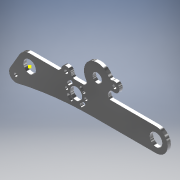
# Autodesk Inventor part: Intake Arm
Saved by Autodesk Inventor 2019.4 (Build 234330000, 330)
## iProperties
Created: 2020-01-28
Part Number: Intake Arm
Material: Aluminum 6061
Document SubType Name: Modeling
Designer: admin
Density: 2.7 g/cm^3
Appearance: Aluminum - Flat
Mass: 119.652 g
Surface Area: 228.427 cm^2
Volume: 44.3155 cm^3
Author: admin
Autodesk Inventor part; units mm, degrees
ref_plane "YZ Plane" through (0, 0, 0) normal (1, 0, 0) x (0, 1, 0)
ref_plane "XZ Plane" through (0, 0, 0) normal (0, 1, 0) x (-1, 0, 0)
ref_plane "XY Plane" through (0, 0, 0) normal (0, 0, 1) x (1, 0, 0)
sketch "Sketch1" plane through (0, 0, 0) normal (0, 0, 1) x (1, 0, 0)
  circle A0 centre (0, 0) radius 9.5
  arc A1 (0, -17.5) -> (0, 17.5) centre (0, 0) ccw construction
  circle A2 centre (190, 0) radius 9.5
  circle A3 centre (-175.4753, -121.2237) radius 88.9 construction
  circle A4 centre (190, 0) radius 41.275 construction
  circle A5 centre (190, 0) radius 28.5 construction
  line L0 (-263.1536, 888.7662) -> (-263.1536, -773.9924) construction
  line L1 (0, 0) -> (190, 0) construction
  arc A6 (190, 17.5) -> (190, -17.5) centre (190, 0) ccw construction
  line L2 (190, 17.5) -> (108.4742, 17.5)
  line L3 (190, -17.5) -> (0, -17.5)
  arc A7 (0, 17.5) -> (-15.1027, 8.8408) centre (0, 0) ccw
  arc A8 (190, -17.5) -> (190, 17.5) centre (190, 0) ccw
  line L4 (0, 0) -> (263.9458, 0) construction
  circle A9 centre (-20.9601, -20.9601) radius 2.5
  circle A10 centre (-20.9601, -20.9601) radius 10
  line L5 (-20.9601, -20.9601) -> (0, 0) construction
  circle A11 centre (-30, 150) radius 2.5 construction
  line L6 (-30, 150) -> (-20.9601, -20.9601) construction
  line L7 (0, -17.5) -> (-14.8786, -28.8983)
  line L8 (-29.5902, -15.9082) -> (-15.1027, 8.8408)
  arc A12 (-15.1027, 8.8408) -> (0, -17.5) centre (0, 0) ccw construction
  line L9 (190, 0) -> (101.6671, 36.3059) construction
  circle A13 centre (70, 0) radius 9
  circle A14 centre (101.6671, 36.3059) radius 7
  line L10 (70, 0) -> (101.6671, 36.3059) construction
  arc A15 (108.4742, 17.5) -> (94.86, 17.5) centre (101.6671, 36.3059) ccw
  arc A16 (94.86, 17.5) -> (108.4742, 17.5) centre (101.6671, 36.3059) ccw construction
  line L11 (94.86, 17.5) -> (0, 17.5)
  line L12 (108.4742, 17.5) -> (94.86, 17.5) construction
  dimension "d0" = 19
  dimension "d1" = 35
  dimension "d4" = 19
  dimension "d5" = 177.8
  dimension "d6" = 82.55
  dimension "d7" = 57
  dimension "d8" = 190
  dimension "d9" = 35
  dimension "d10" = 0
  dimension "d11" = 5
  dimension "d12" = 20
  dimension "d13" = 29.642
  dimension "d14" = 135
  dimension "d15" = 5
  dimension "d16" = 150
  dimension "d17" = 30
  dimension "d18" = 171.1989
  dimension "d20" = 95.503
  dimension "d21" = 18
  dimension "d22" = 14
  dimension "d23" = 48.176
  dimension "d24" = 40
  dimension "d25" = 70
  constraints: 26 end point, 17 centre point, 16 point on circle, 12 tangent, 8 coincident, 1 horizontal, 1 point on line, 1 vertical
  measures "d0" diameter of A0
  measures "d1" diameter of A1
  measures "d4" diameter of A2
  measures "d5" diameter of A3
  measures "d6" diameter of A4
  measures "d7" diameter of A5
  measures "d8" distance of L1.start L1.end
  measures "d9" diameter of A6
  measures "d10" distance between parallel lines of L1 L4
  measures "d11" diameter of A9
  measures "d12" diameter of A10
  measures "d13" distance of L5.start L1.start
  measures "d14" angle of L1 L5
  measures "d15" diameter of A11
  measures "d16" vertical distance of A0.centre L6.start
  measures "d17" horizontal distance of A0.centre L6.start
  measures "d18" distance of L6.start L5.start
  measures "d20" distance of L9.start L9.end
  measures "d21" diameter of A13
  measures "d22" diameter of A14
  measures "d23" distance of L10.start L10.end
  measures "d24" diameter of A15
  measures "d25" distance of point (0, 0) L10.start
extrude "Extrusion1" add sketch "Sketch1" along normal blind 5
fillet "Fillet1" radius 500 1 edges at (0, -17.5, 2.5)
fillet "Fillet2" radius 5 2 edges at (108.4742, 17.5, 2.5) (94.86, 17.5, 2.5)
sketch "Sketch2" plane through (0, 0, 5) normal (0, 0, 1) x (1, 0, 0)
  line L0 (55.5, 0) -> (84.5, 0) construction
  circle A0 centre (70, 0) radius 9 projected
  circle A1 centre (55.5, 0) radius 1.65 construction
  circle A2 centre (84.5, 0) radius 1.65 construction
  circle A3 centre (84.5, 0) radius 2.25
  circle A4 centre (55.5, 0) radius 2.25
  circle A5 centre (70, 0) radius 18.65 construction
  circle A6 centre (70, 0) radius 8.75 projected
  line L1 (84.5009, 6.7619) -> (80.2413, 4.7756) projected
  arc A7 (80.2413, 4.7756) -> (74.7756, 10.2413) centre (70, 0) ccw projected
  line L2 (76.7619, 14.5009) -> (74.7756, 10.2413) projected
  arc A8 (84.5009, 6.7619) -> (76.7619, 14.5009) centre (70, 0) ccw projected
  arc A9 (63.2381, 14.5009) -> (55.4991, 6.7619) centre (70, 0) ccw projected
  line L3 (65.2244, 10.2413) -> (63.2381, 14.5009) projected
  arc A10 (65.2244, 10.2413) -> (59.7587, 4.7756) centre (70, 0) ccw projected
  line L4 (59.7587, 4.7756) -> (55.4991, 6.7619) projected
  line L5 (76.7619, -14.5009) -> (74.7756, -10.2413) projected
  arc A11 (74.7756, -10.2413) -> (80.2413, -4.7756) centre (70, 0) ccw projected
  line L6 (84.5009, -6.7619) -> (80.2413, -4.7756) projected
  arc A12 (76.7619, -14.5009) -> (84.5009, -6.7619) centre (70, 0) ccw projected
  arc A13 (55.4991, -6.7619) -> (63.2381, -14.5009) centre (70, 0) ccw projected
  line L7 (59.7587, -4.7756) -> (55.4991, -6.7619) projected
  arc A14 (59.7587, -4.7756) -> (65.2244, -10.2413) centre (70, 0) ccw projected
  line L8 (65.2244, -10.2413) -> (63.2381, -14.5009) projected
  circle A15 centre (55.5, 0) radius 1.65 projected
  circle A16 centre (84.5, 0) radius 1.65 projected
  point P0 (0, 0)
  point P1 (70, 0)
  dimension "d27" = 29
  dimension "d28" = 4.5
  dimension "d29" = 4.5
  constraints: 3 coincident, 2 centre point, 2 end point, 1 horizontal, 1 midpoint
  measures "d27" distance of L0.start L0.end
  measures "d28" diameter of A3
  measures "d29" diameter of A4
extrude "Extrusion2" cut sketch "Sketch2" against normal through all contours A3 | A4 | L1 A7 L2 A8 | L3 A10 L4 A9 | L5 A11 L6 A12 | L7 A14 L8 A13 | A15 | A16
fillet "Fillet3" radius 2 16 edges at (65.2244, 10.2413, 2.5) (63.2381, 14.5009, 2.5) (55.4991, 6.7619, 2.5) (59.7587, 4.7756, 2.5) (55.4991, -6.7619, 2.5) (63.2381, -14.5009, 2.5) (65.2244, -10.2413, 2.5) (59.7587, -4.7756, 2.5) (74.7756, -10.2413, 2.5) (76.7619, -14.5009, 2.5) (84.5009, -6.7619, 2.5) (80.2413, -4.7756, 2.5) (80.2413, 4.7756, 2.5) (84.5009, 6.7619, 2.5) (74.7756, 10.2413, 2.5) (76.7619, 14.5009, 2.5)
sketch "Sketch3" plane through (0, 0, 5) normal (0, 0, 1) x (1, 0, 0)
  circle A0 centre (127.5093, 37.5) radius 2.75
  circle A1 centre (127.5093, 37.5) radius 7.5
  line L0 (190, 17.5) -> (122.5093, 17.5) projected
  circle A2 centre (55, 21) radius 2.75
  circle A3 centre (55, 21) radius 7.5
  line L1 (80.8249, 17.5) -> (0, 17.5) projected
  point P0 (0, 0)
  dimension "d33" = 5.5
  dimension "d34" = 15
  dimension "d35" = 20
  dimension "d36" = 5
  dimension "d40" = 5.5
  dimension "d41" = 15
  dimension "d42" = 3.5
  dimension "d43" = 55
  constraints: 4 centre point, 2 coincident
  measures "d33" diameter of A0
  measures "d34" diameter of A1
  measures "d35" distance from line of L0 A0.centre
  measures "d36" horizontal distance of L0.end A0.centre
  measures "d40" diameter of A2
  measures "d41" diameter of A3
  measures "d42" distance from line of L1 A2.centre
  measures "d43" horizontal distance of L1.end A2.centre
extrude "Extrusion3" add sketch "Sketch3" against normal up to surface (5 mm away)
fillet "Fillet4" radius 5 4 edges at (121.0365, 41.2886, 2.5) (121.4134, 33.1307, 2.5) (61.6332, 17.5, 2.5) (48.3668, 17.5, 2.5)
sketch "Sketch4" plane through (0, 0, 5) normal (0, 0, 1) x (1, 0, 0)
  point P0 (0, 0)
body "Solid1"
